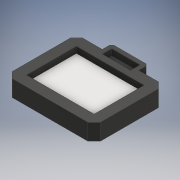
# Autodesk Inventor part: HA11
Saved by Autodesk Inventor 2017 (Build 210142000, 142)
## iProperties
Created: 2019-11-20
Part Number: HA11
Material: ABS Plastic
Document SubType Name: Modeling
Designer: Dell
Density: 1.06 g/cm^3
Appearance: Smooth - Black
Author: Dell
Autodesk Inventor part; units mm, degrees
ref_plane "YZ Plane" through (0, 0, 0) normal (1, 0, 0) x (0, 1, 0)
ref_plane "XZ Plane" through (0, 0, 0) normal (0, 1, 0) x (-1, 0, 0)
ref_plane "XY Plane" through (0, 0, 0) normal (0, 0, 1) x (1, 0, 0)
sketch "Sketch1" plane through (0, 0, 0) normal (0, 0, 1) x (1, 0, 0)
  line L0 (33, 19.0526) -> (33, -19.0526)
  line L1 (33, -19.0526) -> (0, -38.1051)
  line L2 (0, -38.1051) -> (-33, -19.0526)
  line L3 (-33, -19.0526) -> (-33, 19.0526)
  line L4 (-33, 19.0526) -> (0, 38.1051)
  line L5 (0, 38.1051) -> (33, 19.0526)
  line L6 (0, 68.1273) -> (59, 34.0637)
  line L7 (59, 34.0637) -> (59, -34.0637)
  line L8 (59, -34.0637) -> (0, -68.1273)
  line L9 (0, -68.1273) -> (-59, -34.0637)
  line L10 (-59, -34.0637) -> (-59, 34.0637)
  line L11 (-59, 34.0637) -> (0, 68.1273)
  point P0 (0, 0)
  point P1 (0, 0)
  point P2 (0, 0)
  dimension "d0" = 66
  dimension "d1" = 118
  constraints: 24 end point, 2 coincident, 2 vertical alignment, 26 other
  measures "d0" distance between parallel lines of L0 L3
  measures "d1" distance between parallel lines of L7 L10
extrude "Extrusion1" add sketch "Sketch1" along normal blind 13
sketch "Sketch2" plane through (0, 0, 13) normal (0, 0, 1) x (1, 0, 0)
  line L0 (-82.55, 60.96) -> (82.55, 60.96)
  line L1 (82.55, 60.96) -> (82.55, -60.96)
  line L2 (82.55, -60.96) -> (-82.55, -60.96)
  line L3 (-82.55, -60.96) -> (-82.55, 60.96)
  line L4 (107.55, 85.96) -> (-107.55, 85.96)
  line L5 (-107.55, 85.96) -> (-107.55, -85.96)
  line L6 (-107.55, -85.96) -> (107.55, -85.96)
  line L7 (107.55, -85.96) -> (107.55, 85.96)
  point P0 (0, 0)
  point P1 (0, 60.96)
  point P2 (-82.55, 0)
  dimension "d4" = 165.1
  dimension "d5" = 121.92
  dimension "d6" = 25
  constraints: 16 end point, 4 parallel, 2 midpoint, 2 perpendicular, 1 horizontal, 1 horizontal alignment, 1 vertical alignment, 3 other
  measures "d4" distance of L0.start L0.end
  measures "d5" distance of L2.end L0.start
  measures "d6" distance between parallel lines of L0 L4
extrude "Extrusion2" add sketch "Sketch2" along normal blind 40
sketch "Sketch3" plane through (0, 0, 13) normal (0, 0, 1) x (1, 0, 0)
  line L0 (82.55, 60.96) -> (82.55, -60.96) projected
  line L1 (82.55, -60.96) -> (-82.55, -60.96) projected
  line L2 (-82.55, -60.96) -> (-82.55, 60.96) projected
  line L3 (-82.55, 60.96) -> (82.55, 60.96) projected
  line L4 (107.55, 85.96) -> (-107.55, 85.96) projected
  line L5 (-107.55, 85.96) -> (-107.55, -85.96) projected
  line L6 (-107.55, -85.96) -> (107.55, -85.96) projected
  line L7 (107.55, -85.96) -> (107.55, 85.96) projected
  point P0 (0, 0)
extrude "Extrusion3" add sketch "Sketch3" along normal blind 25 contours L0 L1 L2 L3
chamfer "Chamfer1" distance 15 angle 45 4 edges at (107.55, 85.96, 33) (-107.55, 85.96, 33) (-107.55, -85.96, 33) (107.55, -85.96, 33)
sketch "Sketch5" plane through (0, 0, 53) normal (0, 0, 1) x (1, 0, 0)
  line L0 (-34.5, 98.96) -> (34.5, 98.96)
  line L1 (34.5, 98.96) -> (34.5, 75.96)
  line L2 (34.5, 75.96) -> (-34.5, 75.96)
  line L3 (-34.5, 75.96) -> (-34.5, 98.96)
  line L4 (-82.55, 60.96) -> (82.55, 60.96) projected
  line L5 (-44.5, 65.96) -> (44.5, 65.96)
  line L6 (44.5, 65.96) -> (44.5, 108.96)
  line L7 (44.5, 108.96) -> (-44.5, 108.96)
  line L8 (-44.5, 108.96) -> (-44.5, 65.96)
  point P0 (0, 0)
  point P1 (0, 75.96)
  dimension "d16" = 69
  dimension "d17" = 23
  dimension "d18" = 15
  dimension "d19" = 10
  constraints: 16 end point, 4 parallel, 2 perpendicular, 1 horizontal, 1 midpoint, 1 vertical alignment, 3 other
  measures "d16" distance of L1.end L2.end
  measures "d17" distance of L0.end L1.end
  measures "d18" distance between parallel lines of L4 L2
  measures "d19" distance between parallel lines of L5 L2
extrude "Extrusion5" cut sketch "Sketch5" against normal through all contours L0 L1 L2 L3
extrude "Extrusion6" add sketch "Sketch5" against normal up to surface (40 mm away) from surface at 0
sketch "Sketch6" plane through (0, 0, 13) normal (0, 0, -1) x (-1, 0, 0)
  line L0 (-34.5, 98.96) -> (34.5, 98.96) projected
  line L1 (-34.5, 75.96) -> (-34.5, 98.96) projected
  line L2 (34.5, 98.96) -> (34.5, 75.96) projected
  line L3 (34.5, 75.96) -> (-34.5, 75.96) projected
  point P0 (0, 0)
extrude "Extrusion7" add sketch "Sketch6" against normal blind 25
chamfer "Chamfer2" distance 5 angle 45 2 edges at (-44.5, 108.96, 33) (44.5, 108.96, 33)
sketch "Sketch4" plane through (0, 0, 38) normal (0, 0, 1) x (1, 0, 0)
  arc A0 (-11.0008, -6.7698) -> (-71.9286, -8.4622) centre (-38.141, -127.2687) ccw
  arc A1 (-5.9235, 13.5395) -> (-75.3135, 12.2702) centre (-39.1977, -64.7665) ccw
  line L0 (-71.9286, -8.4622) -> (-75.3135, 12.2702)
  line L1 (-5.9235, 13.5395) -> (-11.0008, -6.7698)
  line L2 (0, 0) -> (0, 51.6194) construction
  arc A2 (71.9286, -8.4622) -> (11.0008, -6.7698) centre (38.141, -127.2687) ccw
  arc A3 (75.3135, 12.2702) -> (5.9235, 13.5395) centre (39.1977, -64.7665) ccw
  line L3 (71.9286, -8.4622) -> (75.3135, 12.2702)
  line L4 (5.9235, 13.5395) -> (11.0008, -6.7698)
  arc A4 (-19.0744, -39.0642) -> (63.8895, -28.5788) centre (-4.9616, 182.7337) ccw
  arc A5 (-20.6474, -45.3561) -> (71.9286, -33.1705) centre (-14.0222, 262.0605) ccw
  line L5 (-20.6474, -45.3561) -> (-19.0744, -39.0642)
  line L6 (63.8895, -28.5788) -> (71.9286, -33.1705)
  constraints: 14 end point, 12 point on circle, 6 centre point, 6 symmetric about line, 1 vertical, 2 other
extrude "Extrusion4" [suppressed]
sketch "Sketch7" plane through (0, 0, 38) normal (0, 0, 1) x (1, 0, 0)
  line L0 (-69.7683, 44.5617) -> (-5.8515, 44.5617)
  line L1 (-5.8515, 44.5617) -> (-5.8515, -27.9073)
  line L2 (-5.8515, -27.9073) -> (-69.7683, -27.9073)
  line L3 (-69.7683, -27.9073) -> (-69.7683, 44.5617)
  line L4 (-5.8515, 8.3272) -> (0, 8.3272)
  line L5 (0, 8.3272) -> (0, 0)
  line L6 (0, 0) -> (-5.8515, 0)
  line L7 (-5.8515, 0) -> (-5.8515, 8.3272)
  line L8 (-82.55, -60.96) -> (-82.55, 60.96) projected
  line L9 (-69.7683, 14.8539) -> (-82.55, 14.8539)
  line L10 (-82.55, 14.8539) -> (-82.55, 4.1636)
  line L11 (-82.55, 4.1636) -> (-69.7683, 4.1636)
  line L12 (-69.7683, 4.1636) -> (-69.7683, 14.8539)
  line L13 (69.7683, 44.5617) -> (5.8515, 44.5617)
  line L14 (5.8515, 44.5617) -> (5.8515, -27.9073)
  line L15 (5.8515, -27.9073) -> (69.7683, -27.9073)
  line L16 (69.7683, -27.9073) -> (69.7683, 44.5617)
  line L17 (5.8515, 8.3272) -> (0, 8.3272)
  line L18 (0, 0) -> (5.8515, 0)
  line L19 (5.8515, 0) -> (5.8515, 8.3272)
  line L20 (82.55, -60.96) -> (82.55, 60.96)
  line L21 (69.7683, 14.8539) -> (82.55, 14.8539)
  line L22 (82.55, 14.8539) -> (82.55, 4.1636)
  line L23 (82.55, 4.1636) -> (69.7683, 4.1636)
  line L24 (69.7683, 4.1636) -> (69.7683, 14.8539)
  constraints: 48 end point, 12 symmetric about line, 6 parallel, 4 point on line, 3 horizontal, 3 perpendicular, 1 midpoint
extrude "Extrusion8" [suppressed]
body "Solid1"
